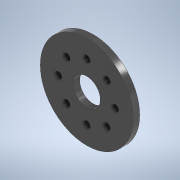
# Autodesk Inventor part: Pulley_base
Saved by Autodesk Inventor 2020 (Build 240168000, 168)
## iProperties
Created: 2019-10-12
Part Number: Pulley_base
Material: Generic
Document SubType Name: Modeling
Designer: ayad493
Density: 1 g/cm^3
Appearance: Dark Gray
Author: ayad493
Autodesk Inventor part; units mm, degrees
ref_plane "YZ Plane" through (0, 0, 0) normal (1, 0, 0) x (0, 1, 0)
ref_plane "XZ Plane" through (0, 0, 0) normal (0, 1, 0) x (-1, 0, 0)
ref_plane "XY Plane" through (0, 0, 0) normal (0, 0, 1) x (1, 0, 0)
sketch "Sketch1" plane through (0, 0, 0) normal (0, 0, 1) x (1, 0, 0)
  circle A0 centre (0, 0) radius 18
  dimension "d0" = 36
  constraints: 1 centre point, 1 coincident
  measures "d0" diameter of A0
extrude "Extrusion1" add sketch "Sketch1" along normal blind 2.5
sketch "Sketch2" plane through (0, 0, 2.5) normal (0, 0, 1) x (1, 0, 0)
  line L0 (0, 0) -> (0, 11)
  circle A0 centre (0, 11) radius 1.25
  circle A1 centre (0, 0) radius 5
  circle A2 centre (7.7782, 7.7782) radius 1.25
  circle A3 centre (11, 0) radius 1.25
  circle A4 centre (7.7782, -7.7782) radius 1.25
  circle A5 centre (0, -11) radius 1.25
  circle A6 centre (-7.7782, -7.7782) radius 1.25
  circle A7 centre (-11, 0) radius 1.25
  circle A8 centre (-7.7782, 7.7782) radius 1.25
  dimension "d3" = 11
  dimension "d4" = 2.5
  dimension "d5" = 10
  dimension "d8" = 360
  constraints: 9 centre point, 2 coincident, 2 end point, 1 vertical, 17 other
  measures "d3" distance of L0.start L0.end
  measures "d4" diameter of A0
  measures "d5" diameter of A1
extrude "Extrusion2" cut sketch "Sketch2" against normal through all
sketch "Sketch3" plane through (0, 0, 2.5) normal (0, 0, 1) x (1, 0, 0)
  circle A0 centre (0, 0) radius 5.25
  dimension "d12" = 10.5
  constraints: 1 centre point, 1 coincident
  measures "d12" diameter of A0
extrude "Extrusion3" cut sketch "Sketch3" against normal through all
sketch "Sketch4" plane through (0, 0, 2.5) normal (0, 0, 1) x (1, 0, 0)
  circle A0 centre (0, 11) radius 1.25 projected
  circle A1 centre (0, 11) radius 1.35
  circle A2 centre (7.7782, 7.7782) radius 1.25 projected
  circle A3 centre (7.7782, 7.7782) radius 1.35
  circle A4 centre (11, 0) radius 1.25 projected
  circle A5 centre (11, 0) radius 1.35
  circle A6 centre (-7.7782, 7.7782) radius 1.25 projected
  circle A7 centre (-7.7782, 7.7782) radius 1.35
  circle A8 centre (-11, 0) radius 1.25 projected
  circle A9 centre (-11, 0) radius 1.35
  circle A10 centre (-7.7782, -7.7782) radius 1.25 projected
  circle A11 centre (-7.7782, -7.7782) radius 1.35
  circle A12 centre (0, -11) radius 1.25 projected
  circle A13 centre (0, -11) radius 1.35
  circle A14 centre (7.7782, -7.7782) radius 1.25 projected
  circle A15 centre (7.7782, -7.7782) radius 1.35
  point P0 (0, 0)
  dimension "d15" = 2.7
  dimension "d16" = 2.7
  dimension "d17" = 2.7
  dimension "d18" = 2.7
  dimension "d19" = 2.7
  dimension "d20" = 2.7
  dimension "d21" = 2.7
  dimension "d22" = 2.7
  constraints: 8 centre point, 8 coincident
  measures "d15" diameter of A1
  measures "d16" diameter of A3
  measures "d17" diameter of A5
  measures "d18" diameter of A7
  measures "d19" diameter of A9
  measures "d20" diameter of A11
  measures "d21" diameter of A13
  measures "d22" diameter of A15
extrude "Extrusion4" cut sketch "Sketch4" against normal blind 10
body "Solid1"
